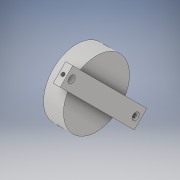
# Autodesk Inventor part: Eraser Interface
Saved by Autodesk Inventor 2019 (Build 230136000, 136)
## iProperties
Created: 2019-06-10
Part Number: Eraser Interface
Material: Generic
Document SubType Name: Modeling
Designer: Matthew XPS
Density: 1 g/cm^3
Appearance: Default
Author: Matthew XPS
Autodesk Inventor part; units mm, degrees
ref_plane "YZ Plane" through (0, 0, 0) normal (1, 0, 0) x (0, 1, 0)
ref_plane "XZ Plane" through (0, 0, 0) normal (0, 1, 0) x (-1, 0, 0)
ref_plane "XY Plane" through (0, 0, 0) normal (0, 0, 1) x (1, 0, 0)
sketch "Sketch2" plane through (0, 0, 0) normal (1, 0, 0) x (0, 1, 0)
  circle A0 centre (0, 0) radius 10
  circle A1 centre (0, 0) radius 22
  line L0 (0, 0) -> (7.0711, -7.0711)
  line L1 (0, 0) -> (10, 0) construction
  circle A2 centre (7.0711, -7.0711) radius 1.5
  line L2 (0, 0) -> (10.8294, 10.8294)
  line L3 (0, 0) -> (15.315, 0) construction
  circle A3 centre (-7.0711, 7.0711) radius 1.5
  dimension "d3" = 20
  dimension "d4" = 44
  dimension "d16" = 10
  dimension "d17" = 45
  dimension "d18" = 3
  dimension "d19" = 45
  constraints: 8 end point, 4 centre point, 3 coincident, 2 equal length, 2 horizontal, 1 symmetric about line, 1 other
  measures "d3" diameter of A0
  measures "d4" diameter of A1
  measures "d16" distance of L0.start L0.end
  measures "d17" angle of L0 L1
  measures "d18" diameter of A2
  measures "d19" angle of L3 L2
extrude "Extrusion1" add sketch "Sketch2" along normal blind 12 contours A2 A0 | A0 L0 A2 | A3 A0 | A0 A3 | A0 A2 L0 | A1
sketch "Sketch4" plane through (0, 0, 0) normal (1, 0, 0) x (0, 0, -1)
  circle A0 centre (0, 0) radius 15.75
  circle A1 centre (15.75, 0) radius 2.55
  dimension "d9" = 31.5
  dimension "d10" = 5.1
  constraints: 1 centre point, 1 coincident, 1 horizontal alignment, 2 other
  measures "d10" diameter of A1
extrude "Extrusion3" cut sketch "Sketch4" along normal blind 30 contours A0 A1 | A0 A1 picked at (14.9184, -0.4924) picked at (16.4994, -0.6699)
sketch "Sketch5" plane through (12, 0, 0) normal (1, 0, 0) x (0, 0, -1)
  circle A0 centre (15.75, 0) radius 2.55 projected
  circle A1 centre (15.75, 0) radius 4.5
  point P0 (0, 0)
  dimension "d20" = 9
  constraints: 1 centre point, 1 coincident
  measures "d20" diameter of A1
extrude "Extrusion4" cut sketch "Sketch5" against normal blind 6
pattern_circular "Circular Pattern1" count 4 over 360 about axis through (-10, 0, 0) along (1, 0, 0) of "Extrusion3", "Extrusion4"
sketch "Sketch6" plane through (12, 0, 0) normal (1, 0, 0) x (0, 0, -1)
  line L0 (0, 0) -> (15.5563, 15.5563)
  line L1 (0, 0) -> (22, 0) construction
  dimension "d23" = 22
  dimension "d24" = 45
  constraints: 4 end point, 1 equal length, 1 horizontal
  measures "d23" distance of L0.start L0.end
  measures "d24" angle of L1 L0
ref_plane "Work Plane1" through (12, 15.5563, -15.5563) normal (0, 0.7071068, -0.7071068) x (-1, 0, 0)
sketch "Sketch7" plane through (12, 15.5563, -15.5563) normal (0, 0.7071068, -0.7071068) x (-1, 0, 0)
  line L0 (0, 22) -> (0, -22) projected
  line L1 (0, 0) -> (12, 0)
  circle A0 centre (6, 0) radius 2.6
  dimension "d25" = 5.2
  constraints: 2 end point, 2 midpoint, 1 centre point, 1 horizontal
  measures "d25" diameter of A0
extrude "Extrusion5" cut sketch "Sketch7" against normal blind 10
ref_plane "Work Plane2" through (12, 0, 0) normal (0, 0.7071068, -0.7071068) x (-1, 0, 0)
mirror "Mirror1" about plane through (12, 0, 0) normal (0, 0.7071068, -0.7071068) of "Extrusion5"
sketch "Sketch8" plane through (0, 0, 0) normal (1, 0, 0) x (0, 1, 0)
  circle A0 centre (-15.75, 0) radius 4.5 projected
  circle A1 centre (0, 15.75) radius 4.5 projected
  circle A2 centre (15.75, 0) radius 4.5 projected
  circle A3 centre (0, -15.75) radius 4.5 projected
  circle A4 centre (0, 0) radius 22 projected
  arc A5 (8.0492, -5.9338) -> (5.9338, -8.0492) centre (7.0711, -7.0711) ccw projected
  arc A6 (-8.0492, 5.9338) -> (5.9338, -8.0492) centre (0, 0) ccw projected
  arc A7 (-8.0492, 5.9338) -> (-5.9338, 8.0492) centre (-7.0711, 7.0711) ccw projected
  arc A8 (8.0492, -5.9338) -> (-5.9338, 8.0492) centre (0, 0) ccw projected
  arc A9 (-7.9786, 5.5166) -> (-5.5166, 7.9786) centre (-7.0711, 7.0711) ccw
  arc A10 (-7.9786, 5.5166) -> (5.5166, -7.9786) centre (0, 0) ccw
  arc A11 (7.9786, -5.5166) -> (5.5166, -7.9786) centre (7.0711, -7.0711) ccw
  arc A12 (7.9786, -5.5166) -> (-5.5166, 7.9786) centre (0, 0) ccw
  dimension "d28" = 0.3
  constraints: 8 point on circle, 4 centre point, 3 other
  measures "d28" radial gap between concentric circles of A8 A12
extrude "Extrusion6" add sketch "Sketch8" along normal blind 12 separate body contours A9 A12 A11 A10
sketch "Sketch9" plane through (0, 0, 0) normal (1, 0, 0) x (0, 1, 0)
  circle A0 centre (0, 0) radius 22 projected
  circle A1 centre (0, 0) radius 28
  circle A2 centre (0, 0) radius 22.25
  dimension "d31" = 6
  dimension "d34" = 0.25
  constraints: 2 centre point
  measures "d31" radial gap between concentric circles of A0 A1
  measures "d34" radial gap between concentric circles of A0 A2
extrude "Extrusion7" add sketch "Sketch9" along normal blind 12 contours A1 bodies 2
sketch "Sketch11" plane through (12, 0, 0) normal (1, 0, 0) x (0, 0, -1)
  line L0 (0, 0) -> (19.799, 19.799)
  circle A0 centre (0, 0) radius 28 projected
  line L1 (0, 0) -> (28, 0) construction
  dimension "d35" = 45
  constraints: 4 end point, 1 equal length, 1 horizontal, 2 other
  measures "d35" angle of L1 L0
ref_plane "Work Plane3" through (12, 19.799, -19.799) normal (0, 0.7071068, -0.7071068) x (-1, 0, 0)
sketch "Sketch12" plane through (12, 19.799, -19.799) normal (0, 0.7071068, -0.7071068) x (-1, 0, 0)
  line L0 (12, 0) -> (0, 0)
  circle A0 centre (6, 0) radius 2.5
  dimension "d36" = 12
  dimension "d37" = 5
  constraints: 2 end point, 1 centre point, 1 horizontal, 1 midpoint
  measures "d36" distance of L0.start L0.end
  measures "d37" diameter of A0
extrude "Extrusion8" cut sketch "Sketch12" against normal blind 10 bodies 2
thread "Thread1" size "M5x0.8" class "6H" standard "ANSI Metric M Profile" full length
mirror "Mirror2" about plane through (12, 0, 0) normal (0, 0.7071068, -0.7071068) of "Extrusion8" bodies 2
sketch "Sketch13" plane through (12, 0, 0) normal (1, 0, 0) x (0, 0, -1)
  circle A0 centre (0, 0) radius 28 projected
  circle A1 centre (0, 0) radius 28 projected
extrude "Extrusion9" add sketch "Sketch13" along normal blind 5 bodies 2
sketch "Sketch22" plane through (17, 0, 0) normal (1, 0, 0) x (0, 0, -1)
  line L0 (36.7696, -26.163) -> (-26.163, 36.7696)
  line L1 (-26.163, 36.7696) -> (-36.7696, 26.163)
  line L2 (-36.7696, 26.163) -> (26.163, -36.7696)
  line L3 (26.163, -36.7696) -> (36.7696, -26.163)
  line L4 (36.7696, -26.163) -> (-36.7696, 26.163) construction
  line L5 (-26.163, 36.7696) -> (26.163, -36.7696) construction
  line L6 (36.7696, -26.163) -> (125.7696, -26.163) construction
  point P0 (0, 0)
  dimension "d73" = 89
  dimension "d74" = 225
  dimension "d75" = 15
  constraints: 14 end point, 2 midpoint, 2 parallel, 1 equal length, 1 horizontal, 1 perpendicular
  measures "d73" distance of L0.start L0.end
  measures "d75" distance of L1.end L0.end
extrude "Extrusion14" add sketch "Sketch22" along normal blind 6 bodies 2
sketch "Sketch23" plane through (23, 0, 0) normal (1, 0, 0) x (0, 0, -1)
  line L0 (-26.163, 36.7696) -> (-36.7696, 26.163) projected
  line L1 (-31.4663, 31.4663) -> (-27.2236, 27.2236)
  line L2 (-31.4663, 31.4663) -> (-25.4663, 31.4663) construction
  circle A0 centre (-27.2236, 27.2236) radius 3.05
  point P0 (0, 0)
  dimension "d78" = 6
  dimension "d79" = 45
  dimension "d80" = 6.1
  constraints: 4 end point, 1 centre point, 1 coincident, 1 equal length, 1 horizontal, 1 midpoint, 1 perpendicular
  measures "d78" distance of L1.start L1.end
  measures "d79" angle of L1 L2
  measures "d80" diameter of A0
extrude "Extrusion15" cut sketch "Sketch23" against normal blind 5.2 bodies 2
sketch "Sketch24" plane through (17, 26.163, 36.7696) normal (0, 0.7071068, 0.7071068) x (1, 0, 0)
  line L0 (0, 0) -> (6, 0) projected
  line L1 (3, 0) -> (3, 15)
  line L2 (0, 15) -> (6, 15) projected
  circle A0 centre (3, 7.5) radius 1.5
  point P0 (-17, 7.5)
  dimension "d83" = 3
  constraints: 3 midpoint, 2 end point, 1 centre point
  measures "d83" diameter of A0
extrude "Extrusion16" cut sketch "Sketch24" against normal blind 5.2 bodies 2
thread "Thread3" size "M3x0.5" class "6H" standard "ANSI Metric M Profile" full length
ref_plane "Work Plane5" through (17, -5.3033, 5.3033) normal (0, 0.7071068, 0.7071068) x (1, 0, 0)
mirror "Mirror3" about plane through (17, -5.3033, 5.3033) normal (0, 0.7071068, 0.7071068) of "Extrusion15", "Extrusion16" bodies 2
body "Solid1"
body "Solid2"
